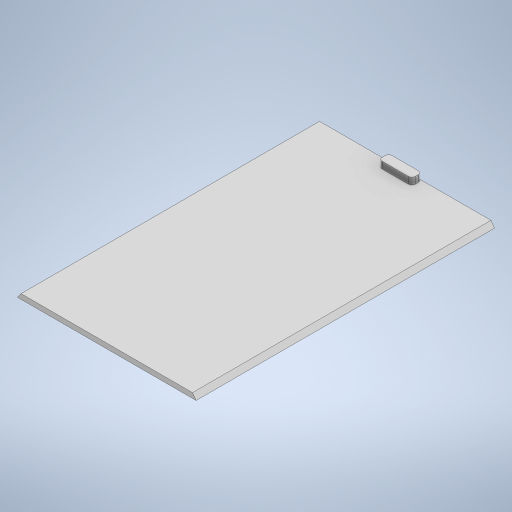
# Autodesk Inventor part: cover2
Saved by Autodesk Inventor 2023 (Build 270158000, 158)
## iProperties
Created: 2023-03-10
Part Number: cover2
Material: Типовые
Document SubType Name: Modeling
Designer: Josh
Density: 1 g/cm^3
Appearance: По умолчанию
Author: Josh
Autodesk Inventor part; units mm, degrees
ref_plane "YZ Plane" through (0, 0, 0) normal (1, 0, 0) x (0, 1, 0)
ref_plane "XZ Plane" through (0, 0, 0) normal (0, 1, 0) x (-1, 0, 0)
ref_plane "XY Plane" through (0, 0, 0) normal (0, 0, 1) x (1, 0, 0)
sketch "Эскиз1" plane through (0, 0, 0) normal (0, 0, 1) x (1, 0, 0)
  line L0 (0, -0.6) -> (0, 3.6) projected
  line L1 (0, 0) -> (0, 3)
  line L2 (-24.75, 3) -> (24.75, 3)
  line L3 (-26.95, 0) -> (26.95, 0)
  line L4 (-24.75, 3) -> (-26.95, 0)
  line L5 (24.75, 3) -> (26.95, 0)
  line L6 (-25.85, 1.5) -> (25.85, 1.5)
  dimension "d1" = 3
  dimension "d3" = 49.5
  dimension "d4" = 53.9
  constraints: 12 end point, 4 midpoint, 2 horizontal, 1 point on line
  measures "d1" distance of L1.end L1.start
  measures "d3" distance of L2.start L2.end
  measures "d4" distance of L3.start L3.end
extrude "Выдавливание1" add sketch "Эскиз1" along normal blind 90 contours L3 L4 L6 L0 | L0 L6 L5 L3
sketch "Эскиз2" plane through (-25.85, 1.5, 0) normal (0, 1, 0) x (1, 0, 0)
  line L0 (-1.1, 0) -> (52.8, 0) projected
  line L1 (20.85, 0) -> (30.85, 0)
  line L2 (30.85, 0) -> (30.85, -3)
  line L3 (30.85, -3) -> (20.85, -3)
  line L4 (20.85, -3) -> (20.85, 0)
  line L5 (25.85, 18) -> (25.85, -108) projected
  point P0 (25.85, 0)
  dimension "d7" = 10
  dimension "d8" = 3
  constraints: 8 end point, 2 parallel, 1 horizontal, 1 perpendicular, 1 point on line, 1 other
  measures "d7" distance between parallel lines of L2 L4
  measures "d8" distance between parallel lines of L0 L3
extrude "Выдавливание2" add sketch "Эскиз2" along normal blind 2
fillet "Сопряжение1" radius 1 4 edges at (5, 2.5, 3) (5, 2.5, 0) (-5, 2.5, 3) (-5, 2.5, 0)
